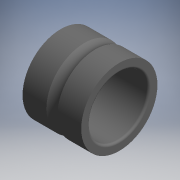
# Autodesk Inventor part: 684AZZ Inner Ring
Saved by Autodesk Inventor 2017.3 (Build 213256000, 256)
## iProperties
Part Number: 684AZZ Inner Ring
Material: Generic
Catalog Web Link: www.cadenas.de
Description: shielde_type_zz_zzs_IR-
Vendor: NSK_RB
Document SubType Name: Modeling
Designer: partserver
Manufacturer: NSK_RB
Mass: 0.0337461 g
Surface Area: 1.31602 cm^2
Volume: 0.0337461 cm^3
Density: 1 g/cm^3
Appearance: PSOLRGB-128-128-128
Category: PARTsolutions
Company: NSK_RB
Title: 684AZZ Inner Ring
Author: Cadenas PARTsolutions
PSOL_IDENT_0: {$CADENAS_DATA\23d-libs\nsk_rb\roller_bearings\deep_groove_bb\exstra_small_miniatur_bb\metric_design
PSOL_IDENT_1: \shielded_type_zz_zzs_ir.prj},191 {VTYP=3D},{NB=684AZZ Inner Ring},{LINA=684AZZ Inner Ring},{NN=shie
PSOL_IDENT_2: lde_type_zz_zzs_IR},{DATE=30.03.2022 01:55:07},{GEOMDATE=04.01.2008 00:00:00},{VERSION=},{LINEID=220
PSOL_IDENT_3: },{WBVAR=},{WBNUMERIC=}  {NB=684AZZ Inner Ring},{LINA=684AZZ Inner Ring},{KT=DUMMY},{IDNR=},{STAN=St
PSOL_IDENT_4: andard},{ORDER=684AZZ},{SD=4.0},{X=4.0},{DI1=5.20},{DI2=5.20},{SDE1=7.50},{SDE2=8.10},{D=9},{DD=9},{
PSOL_IDENT_5: B=0.0},{B1=4.0},{R=0.00},{R1=0.15},{CR1=640},{COR1=225},{CR2=65},{COR2=23.0},{LG=53000},{LO=63000},{
PSOL_IDENT_6: DA=0.0},{DB=5.2},{DA1=0.0},{DB1=8.1},{RA=0.00},{RB=0.10},{MASS=1.01},{SC=1},{N=10}
NB: 684AZZ Inner Ring
NN: shielde_type_zz_zzs_IR
NBSYN: $ORDER. Inner Ring
LINA: 684AZZ Inner Ring
CATALOG: NSK Rolling Bearing
STAN: Standard
ORDER: 684AZZ
SD: 4
X: 4
DI1: 5.2
DI2: 5.2
SDE1: 7.5
SDE2: 8.1
D: 9
DD: 9
B: 0
B1: 4
R: 0
R1: 0.15
CR1: 640
COR1: 225
CR2: 65
COR2: 23
LG: 53000
LO: 63000
DA: 0
DB: 5.2
DA1: 0
DB1: 8.1
RA: 0
RB: 0.1
MASS: 1.01
SC: 1
SUPPLIER: NSK_RB
ARTICLENO: 684AZZ Inner Ring
BOMINFO: 684AZZ Inner Ring
CREATOR: CADENAS GmbH
Autodesk Inventor part; units mm, degrees
sketch "Sketch_1" plane through (0, 0, 0) normal (0, 0, 1) x (1, 0, 0)
  line L0 (4, 0) -> (0, 0)
  arc A0 (0, 2.15) -> (0.15, 2) centre (0.15, 2.15) ccw
  line L1 (0.15, 2) -> (3.85, 2)
  arc A1 (3.85, 2) -> (4, 2.15) centre (3.85, 2.15) ccw
  line L2 (4, 2.15) -> (4, 2.6)
  line L3 (4, 2.6) -> (2.3742, 2.6)
  arc A2 (1.6258, 2.6) -> (2.3742, 2.6) centre (2, 3.25) ccw
  line L4 (1.6258, 2.6) -> (0, 2.6)
  line L5 (0, 2.6) -> (0, 2.15)
  constraints: 12 end point, 6 point on circle, 3 centre point
revolve "Revolution1" add sketch "Sketch_1" angle 360 about axis through (4, 0, 0) along (1, 0, 0)
ref_plane "ip_st_ir_1_1_XY" through (2, 3.25, 0) normal (1, 0, 0) x (0, 0, -1)
ref_plane "ip_st_ir_1_1_YZ" through (2, 3.25, 0) normal (0, 0, -1) x (0, 1, 0)
ref_plane "ip_st_ir_1_1_ZX" through (2, 3.25, 0) normal (0, 1, 0) x (1, 0, 0)
ref_plane "ip_st_ir_1_10_XY" through (2, 2.6293, -1.9103) normal (1, 0, 0) x (0, 0, -1)
ref_plane "ip_st_ir_1_10_YZ" through (2, 2.6293, -1.9103) normal (0, 0, -1) x (0, 1, 0)
ref_plane "ip_st_ir_1_10_ZX" through (2, 2.6293, -1.9103) normal (0, 1, 0) x (1, 0, 0)
ref_plane "ip_st_ir_1_2_XY" through (2, 2.6293, 1.9103) normal (1, 0, 0) x (0, 0, -1)
ref_plane "ip_st_ir_1_2_YZ" through (2, 2.6293, 1.9103) normal (0, 0, -1) x (0, 1, 0)
ref_plane "ip_st_ir_1_2_ZX" through (2, 2.6293, 1.9103) normal (0, 1, 0) x (1, 0, 0)
ref_plane "ip_st_ir_1_3_XY" through (2, 1.0043, 3.0909) normal (1, 0, 0) x (0, 0, -1)
ref_plane "ip_st_ir_1_3_YZ" through (2, 1.0043, 3.0909) normal (0, 0, -1) x (0, 1, 0)
ref_plane "ip_st_ir_1_3_ZX" through (2, 1.0043, 3.0909) normal (0, 1, 0) x (1, 0, 0)
ref_plane "ip_st_ir_1_4_XY" through (2, -1.0043, 3.0909) normal (1, 0, 0) x (0, 0, -1)
ref_plane "ip_st_ir_1_4_YZ" through (2, -1.0043, 3.0909) normal (0, 0, -1) x (0, 1, 0)
ref_plane "ip_st_ir_1_4_ZX" through (2, -1.0043, 3.0909) normal (0, 1, 0) x (1, 0, 0)
ref_plane "ip_st_ir_1_5_XY" through (2, -2.6293, 1.9103) normal (1, 0, 0) x (0, 0, -1)
ref_plane "ip_st_ir_1_5_YZ" through (2, -2.6293, 1.9103) normal (0, 0, -1) x (0, 1, 0)
ref_plane "ip_st_ir_1_5_ZX" through (2, -2.6293, 1.9103) normal (0, 1, 0) x (1, 0, 0)
ref_plane "ip_st_ir_1_6_XY" through (2, -3.25, 0) normal (1, 0, 0) x (0, 0, -1)
ref_plane "ip_st_ir_1_6_YZ" through (2, -3.25, 0) normal (0, 0, -1) x (0, 1, 0)
ref_plane "ip_st_ir_1_6_ZX" through (2, -3.25, 0) normal (0, 1, 0) x (1, 0, 0)
ref_plane "ip_st_ir_1_7_XY" through (2, -2.6293, -1.9103) normal (1, 0, 0) x (0, 0, -1)
ref_plane "ip_st_ir_1_7_YZ" through (2, -2.6293, -1.9103) normal (0, 0, -1) x (0, 1, 0)
ref_plane "ip_st_ir_1_7_ZX" through (2, -2.6293, -1.9103) normal (0, 1, 0) x (1, 0, 0)
ref_plane "ip_st_ir_1_8_XY" through (2, -1.0043, -3.0909) normal (1, 0, 0) x (0, 0, -1)
ref_plane "ip_st_ir_1_8_YZ" through (2, -1.0043, -3.0909) normal (0, 0, -1) x (0, 1, 0)
ref_plane "ip_st_ir_1_8_ZX" through (2, -1.0043, -3.0909) normal (0, 1, 0) x (1, 0, 0)
ref_plane "ip_st_ir_1_9_XY" through (2, 1.0043, -3.0909) normal (1, 0, 0) x (0, 0, -1)
ref_plane "ip_st_ir_1_9_YZ" through (2, 1.0043, -3.0909) normal (0, 0, -1) x (0, 1, 0)
ref_plane "ip_st_ir_1_9_ZX" through (2, 1.0043, -3.0909) normal (0, 1, 0) x (1, 0, 0)
ref_plane "ip_st_ir_1a_XY" through (0, 0, 0) normal (1, 0, 0) x (0, 0, -1)
ref_plane "ip_st_ir_1a_YZ" through (0, 0, 0) normal (0, 0, -1) x (0, 1, 0)
ref_plane "ip_st_ir_1a_ZX" through (0, 0, 0) normal (0, 1, 0) x (1, 0, 0)
ref_plane "ip_st_ir_2a_XY" through (0.2656, 0, 0) normal (1, 0, 0) x (0, 0, -1)
ref_plane "ip_st_ir_2a_YZ" through (0.2656, 0, 0) normal (0, 0, -1) x (0, 1, 0)
ref_plane "ip_st_ir_2a_ZX" through (0.2656, 0, 0) normal (0, 1, 0) x (1, 0, 0)
body "Solid1"
